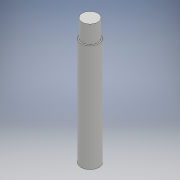
# Autodesk Inventor part: handAdaptation
Saved by Autodesk Inventor 2017 (Build 210142000, 142)
## iProperties
Created: 2017-08-20
Part Number: handAdaptation
Material: Generic
Document SubType Name: Modeling
Designer: Bardo91
Density: 1 g/cm^3
Appearance: Default
Author: Bardo91
Autodesk Inventor part; units mm, degrees
ref_plane "YZ Plane" through (0, 0, 0) normal (1, 0, 0) x (0, 1, 0)
ref_plane "XZ Plane" through (0, 0, 0) normal (0, 1, 0) x (-1, 0, 0)
ref_plane "XY Plane" through (0, 0, 0) normal (0, 0, 1) x (1, 0, 0)
sketch "Sketch1" plane through (0, 0, 0) normal (0, 0, 1) x (1, 0, 0)
  circle A0 centre (0, 0) radius 5
  dimension "d0" = 10
  constraints: 1 centre point, 1 coincident
  measures "d0" diameter of A0
extrude "Extrusion1" add sketch "Sketch1" along normal blind 60
sketch "Sketch2" plane through (0, 0, 60) normal (0, 0, 1) x (1, 0, 0)
  circle A0 centre (0, 0) radius 4.375
  dimension "d3" = 8.75
  constraints: 1 centre point, 1 coincident
  measures "d3" diameter of A0
extrude "Extrusion2" add sketch "Sketch2" along normal blind 10
body "Solid1"
